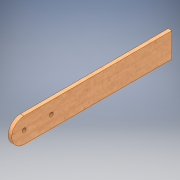
# Autodesk Inventor part: Część4
Saved by Autodesk Inventor 2017 (Build 210142000, 142)
## iProperties
Created: 2017-05-17
Part Number: Część4
Material: Drewno (wiśnia)
Document SubType Name: Modeling
Designer: Damian
Density: 0.63 g/cm^3
Appearance: Wiśnia — naturalna — niski połysk
Author: Damian
Autodesk Inventor part; units mm, degrees
ref_plane "YZ Plane" through (0, 0, 0) normal (1, 0, 0) x (0, 1, 0)
ref_plane "XZ Plane" through (0, 0, 0) normal (0, 1, 0) x (-1, 0, 0)
ref_plane "XY Plane" through (0, 0, 0) normal (0, 0, 1) x (1, 0, 0)
sketch "Szkic1" plane through (0, 0, 0) normal (1, 0, 0) x (0, 1, 0)
  line L0 (10, 0) -> (130, 0)
  line L1 (130, 0) -> (130, 20)
  line L2 (130, 20) -> (10, 20)
  line L3 (0, 10) -> (0, 10)
  arc A0 (0, 10) -> (10, 0) centre (10, 10) ccw
  arc A1 (10, 20) -> (0, 10) centre (10, 10) ccw
  circle A2 centre (32, 10) radius 1.6
  point P0 (0, 0)
  point P1 (0, 20)
  dimension "d0" = 20
  dimension "d2" = 10
  dimension "d12" = 120
  dimension "d13" = 32
  dimension "d14" = 3.2
  constraints: 8 end point, 4 point on circle, 4 point on line, 4 tangent, 3 centre point, 2 parallel, 1 coincident, 1 concentric, 1 horizontal, 1 perpendicular
  measures "d0" distance of L0.end L1.end
  measures "d2" radius of A0
  measures "d12" distance from line of L1 A0.centre
  measures "d13" distance of L3.end point (32, 10)
  measures "d14" diameter of A2
extrude "Wyciągnięcie proste1" add sketch "Szkic1" along normal blind 3 contours A0 A1 L2 L1 L0 | A2
sketch "Szkic2" plane through (3, 0, 0) normal (1, 0, 0) x (0, 0, -1)
  arc A0 (-20, 10) -> (0, 10) centre (-10, 10) ccw projected
  point P0 (0, 0)
  constraints: 1 coincident
hole "Otwór1" at (3, 10, 10) direction (-1, 0, 0) diameter 3.2 end through all
sketch "Szkic3" plane through (3, 0, 0) normal (1, 0, 0) x (0, 0, -1)
  point P0 (0, 0)
  point P1 (-10, 32)
  dimension "d15" = 32
  measures "d15" vertical distance of point (0, 0) point (-10, 32)
hole "Otwór2" at (3, 32, 10) direction (-1, 0, 0) diameter 3.2 end through all
